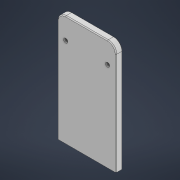
# Autodesk Inventor part: motorHolder_stator
Saved by Autodesk Inventor 2021 (Build 250183000, 183)
## iProperties
Created: 2021-06-20
Part Number: motorHolder_stator
Material: Generic
Document SubType Name: Modeling
Designer: Watchdog
Density: 1 g/cm^3
Appearance: Default
Author: Watchdog
Autodesk Inventor part; units mm, degrees
ref_plane "YZ Plane" through (0, 0, 0) normal (1, 0, 0) x (0, 1, 0)
ref_plane "XZ Plane" through (0, 0, 0) normal (0, 1, 0) x (-1, 0, 0)
ref_plane "XY Plane" through (0, 0, 0) normal (0, 0, 1) x (1, 0, 0)
sketch "Sketch1" plane through (0, 0, 0) normal (0, 0, 1) x (1, 0, 0)
  line L0 (-35, 0) -> (35, 0)
  line L1 (35, 0) -> (35, 132)
  line L2 (35, 132) -> (-35, 132)
  line L3 (-35, 132) -> (-35, 0)
  point P0 (0, 0)
  dimension "d0" = 70
  dimension "d1" = 35
  dimension "d2" = 132
  constraints: 8 end point, 2 parallel, 1 horizontal, 1 midpoint, 1 perpendicular
  measures "d0" distance between parallel lines of L1 L3
  measures "d1" distance from line of point (0, 0) L3
  measures "d2" distance between parallel lines of L0 L2
extrude "Extrusion1" add sketch "Sketch1" along normal blind 8
fillet "Fillet1" radius 10 2 edges at (-35, 132, 4) (35, 132, 4)
sketch "Sketch2" plane through (0, 0, 8) normal (0, 0, 1) x (1, 0, 0)
  line L0 (35, 0) -> (35, 122) projected
  line L1 (-35, 122) -> (-35, 0) projected
  line L2 (25, 132) -> (-25, 132) projected
  line L3 (-35, 0) -> (35, 0) projected
  point P0 (0, 0)
  point P1 (-25, 106.6)
  point P2 (25, 106.6)
  dimension "d6" = 70
  dimension "d9" = 50
  dimension "d10" = 0
  dimension "d11" = 10
  dimension "d13" = 106.6
  measures "d6" distance between parallel lines of L0 L1
  measures "d9" distance of point (25, 106.6) point (-25, 106.6)
  measures "d10" vertical distance of point (25, 106.6) point (-25, 106.6)
  measures "d11" distance from line of L1 point (-25, 106.6)
  measures "d13" distance from line of point (25, 106.6) L3
hole "Hole1" at (-25, 106.6, 8) at (25, 106.6, 8) direction (0, 0, -1) diameter 5 depth 8
chamfer "Chamfer1" distance 1 angle 45 10 edges at (0, 132, 8) (-32.0711, 129.0711, 8) (-35, 61, 8) (32.0711, 129.0711, 8) (35, 61, 8) (0, 132, 0) (-32.0711, 129.0711, 0) (-35, 61, 0) (32.0711, 129.0711, 0) (35, 61, 0)
equation "\"d1\" = 0.5 * d0"
equation "\"d11\" = -0.5 * d9 + 0.5 * d6"
body "Solid1"
